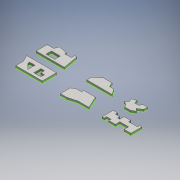
# Autodesk Inventor part: 240329_직선연습
Saved by Autodesk Inventor 2016 (Build 200138000, 138)
## iProperties
Created: 2024-03-29
Part Number: 240329_직선연습
Material: 일반
Document SubType Name: Modeling
Designer: pc
Density: 1 g/cm^3
Appearance: 기본값
Author: pc
Autodesk Inventor part; units mm, degrees
ref_plane "YZ Plane" through (0, 0, 0) normal (1, 0, 0) x (0, 1, 0)
ref_plane "XZ Plane" through (0, 0, 0) normal (0, 1, 0) x (-1, 0, 0)
ref_plane "XY Plane" through (0, 0, 0) normal (0, 0, 1) x (1, 0, 0)
sketch "스케치1" plane through (0, 0, 0) normal (0, 0, 1) x (1, 0, 0)
  line L0 (-17.9838, 5.9383) -> (12.0162, 5.9383)
  line L1 (-17.9838, 5.9383) -> (-17.9838, -44.0617)
  line L2 (-17.9838, -44.0617) -> (110.0162, -44.0617)
  line L3 (110.0162, -44.0617) -> (97.8609, 24.8748)
  line L4 (97.8609, 24.8748) -> (87.8609, 24.8748)
  line L5 (87.8609, 24.8748) -> (87.8609, 9.8748)
  line L6 (87.8609, 9.8748) -> (57.8609, 9.8748)
  line L7 (57.8609, 9.8748) -> (57.8609, 17.8748)
  line L8 (57.8609, 17.8748) -> (18.4685, 24.8207)
  line L9 (18.4685, 24.8207) -> (12.0162, 5.9383)
  line L10 (17.0386, -9.366) -> (57.0386, -9.366)
  line L11 (57.0386, -9.366) -> (57.0386, -34.366)
  line L12 (57.0386, -34.366) -> (17.0386, -34.366)
  line L13 (17.0386, -34.366) -> (17.0386, -9.366)
  line L14 (-21.4983, -83.6189) -> (113.5017, -83.6189)
  line L15 (113.5017, -83.6189) -> (113.5017, -147.6189)
  line L16 (113.5017, -147.6189) -> (-6.4983, -147.6189)
  line L17 (-6.4983, -147.6189) -> (-6.4983, -112.6189)
  line L18 (-6.4983, -112.6189) -> (-21.4983, -83.6189)
  line L19 (11.4782, -102.6977) -> (11.4782, -110.6977)
  line L20 (11.4782, -102.6977) -> (35.4782, -102.6977)
  line L21 (35.4782, -102.6977) -> (35.4782, -134.6977)
  line L22 (35.4782, -134.6977) -> (11.4782, -110.6977)
  line L23 (62.4782, -102.6977) -> (62.4782, -134.6977)
  line L24 (62.4782, -134.6977) -> (94.4782, -134.6977)
  line L25 (94.4782, -134.6977) -> (94.4782, -118.6977)
  line L26 (94.4782, -118.6977) -> (78.4782, -118.6977)
  line L27 (78.4782, -118.6977) -> (78.4782, -102.6977)
  line L28 (78.4782, -102.6977) -> (62.4782, -102.6977)
  line L29 (210.3042, -22.2898) -> (210.3042, -42.2898)
  line L30 (210.3042, -42.2898) -> (325.3042, -42.2898)
  line L31 (325.3042, -42.2898) -> (308.521, -17.4237)
  line L32 (308.521, -17.4237) -> (288.521, -17.4237)
  line L33 (288.521, -17.4237) -> (279.9747, 2.7102)
  line L34 (279.9747, 2.7102) -> (240.098, 2.7102)
  line L35 (240.098, 2.7102) -> (210.3042, -22.2898)
  line L36 (243.03, -90.9913) -> (298.03, -90.9913)
  line L37 (298.03, -90.9913) -> (323.3871, -145.3698)
  line L38 (323.3871, -145.3698) -> (273.3871, -145.3698)
  line L39 (273.3871, -145.3698) -> (234.8117, -156.4311)
  line L40 (234.8117, -156.4311) -> (204.822, -156.4311)
  line L41 (204.822, -156.4311) -> (204.822, -111.4311)
  line L42 (204.822, -111.4311) -> (222.1425, -101.4311)
  line L43 (222.1425, -101.4311) -> (247.0375, -101.4311)
  line L44 (247.0375, -101.4311) -> (243.03, -90.9913)
  line L45 (391.7462, -29.9278) -> (380.8188, -42.9505)
  line L46 (380.8188, -42.9505) -> (394.4134, -49.2898)
  line L47 (394.4134, -49.2898) -> (404.1642, -63.2154)
  line L48 (404.1642, -63.2154) -> (429.1642, -63.2154)
  line L49 (429.1642, -63.2154) -> (446.4847, -53.2154)
  line L50 (391.7462, -29.9278) -> (386.6159, -15.8324)
  line L51 (391.7462, -29.9278) -> (406.7462, -29.9278) construction
  line L52 (386.6159, -15.8324) -> (405.4097, -8.992)
  line L53 (405.4097, -8.992) -> (411.2241, -24.9667)
  line L54 (455.4729, -12.2341) -> (435.4737, -12.0471)
  line L55 (435.4737, -12.0471) -> (427.8526, -24.9667)
  line L56 (411.2241, -24.9667) -> (427.8526, -24.9667)
  line L57 (455.4729, -12.2341) -> (455.4729, -29.2341)
  line L58 (455.4729, -29.2341) -> (434.9941, -43.5735)
  line L59 (434.9941, -43.5735) -> (446.4847, -53.2154)
  line L60 (390.4902, -102.3026) -> (410.4902, -102.3026)
  line L61 (410.4902, -102.3026) -> (410.4902, -112.3026)
  line L62 (410.4902, -112.3026) -> (430.4902, -112.3026)
  line L63 (430.4902, -112.3026) -> (430.4902, -122.3026)
  line L64 (430.4902, -122.3026) -> (440.4902, -122.3026)
  line L65 (440.4902, -122.3026) -> (440.4902, -102.3026)
  line L66 (440.4902, -102.3026) -> (470.4902, -102.3026)
  line L67 (470.4902, -102.3026) -> (470.4902, -112.3026)
  line L68 (470.4902, -112.3026) -> (510.4902, -112.3026)
  line L69 (510.4902, -112.3026) -> (510.4902, -102.3026)
  line L70 (510.4902, -102.3026) -> (520.4902, -102.3026)
  line L71 (520.4902, -102.3026) -> (520.4902, -152.3026)
  line L72 (390.4902, -102.3026) -> (390.4902, -152.3026)
  line L73 (390.4902, -152.3026) -> (400.4902, -152.3026)
  line L74 (400.4902, -152.3026) -> (400.4902, -142.3026)
  line L75 (400.4902, -142.3026) -> (420.4902, -142.3026)
  line L76 (420.4902, -142.3026) -> (420.4902, -152.3026)
  line L77 (420.4902, -152.3026) -> (450.4902, -152.3026)
  line L78 (450.4902, -152.3026) -> (450.4902, -132.3026)
  line L79 (450.4902, -132.3026) -> (490.4902, -132.3026)
  line L80 (490.4902, -132.3026) -> (490.4902, -152.3026)
  line L81 (490.4902, -152.3026) -> (520.4902, -152.3026)
  point P0 (0, 0)
  dimension "d0" = 30
  dimension "d1" = 50
  dimension "d2" = 128
  dimension "d3" = 70
  dimension "d4" = 80
  dimension "d5" = 10
  dimension "d6" = 15
  dimension "d7" = 30
  dimension "d8" = 8
  dimension "d9" = 40
  dimension "d10" = 100
  dimension "d11" = 40
  dimension "d12" = 25
  dimension "d13" = 135
  dimension "d14" = 64
  dimension "d15" = 120
  dimension "d16" = 35
  dimension "d17" = 8
  dimension "d18" = 24
  dimension "d19" = 32
  dimension "d20" = 32
  dimension "d21" = 16
  dimension "d22" = 16
  dimension "d23" = 27
  dimension "d28" = 20
  dimension "d29" = 115
  dimension "d30" = 30
  dimension "d31" = 20
  dimension "d32" = 67
  dimension "d33" = 50
  dimension "d34" = 45
  dimension "d35" = 55
  dimension "d36" = 60
  dimension "d37" = 50
  dimension "d38" = 65
  dimension "d39" = 40.13
  dimension "d40" = 16
  dimension "d41" = 45
  dimension "d42" = 20
  dimension "d43" = 120
  dimension "d44" = 69
  dimension "d56" = 17
  dimension "d58" = 15
  dimension "d59" = 75
  dimension "d60" = 17
  dimension "d61" = 150
  dimension "d62" = 25
  dimension "d63" = 20
  dimension "d64" = 150
  dimension "d77" = 125
  dimension "d78" = 15
  dimension "d80" = 20
  dimension "d81" = 17
  dimension "d82" = 20
  dimension "d83" = 15
  dimension "d84" = 120
  dimension "d85" = 120
  dimension "d87" = 90
  dimension "d88" = 90
  dimension "d97" = 17
  dimension "d98" = 25
  dimension "d99" = 55
  dimension "d100" = 75
  dimension "d103" = 20
  constraints: 164 end point, 33 perpendicular, 10 horizontal, 8 vertical, 7 point on line, 4 parallel
  measures "d0" distance of L0.start L0.end
  measures "d1" distance of L0.start L1.end
  measures "d2" distance of L1.end L2.end
  measures "d3" distance of L2.end L3.end
  measures "d4" angle of L3 L2
  measures "d5" distance of L3.end L4.end
  measures "d6" distance of L4.end L5.end
  measures "d7" distance of L5.end L6.end
  measures "d8" distance of L6.end L7.end
  measures "d9" distance of L7.end L8.end
  measures "d10" angle of L8 L7
  measures "d11" distance of L11.end L12.end
  measures "d12" distance of L10.end L11.end
  measures "d13" distance of L14.start L14.end
  measures "d14" distance of L14.end L15.end
  measures "d15" distance of L15.end L16.end
  measures "d16" distance of L16.end L17.end
  measures "d17" distance of L19.start L19.end
  measures "d18" distance of L19.start L20.end
  measures "d19" distance of L20.end L21.end
  measures "d20" distance of L23.end L24.end
  measures "d21" distance of L25.end L26.end
  measures "d22" distance of L26.end L27.end
  measures "d23" distance of L23.start L20.end
  measures "d28" distance of L29.start L29.end
  measures "d29" distance of L29.end L30.end
  measures "d30" distance of L30.end L31.end
  measures "d31" distance of L31.end L32.end
  measures "d32" angle of L32 L33
  measures "d33" angle of L29 L35
  measures "d34" distance between parallel lines of L30 L34
  measures "d35" distance of L36.start L36.end
  measures "d36" distance of L36.end L37.end
  measures "d37" distance of L37.end L38.end
  measures "d38" angle of L37 L38
  measures "d39" distance of L38.end L39.end
  measures "d40" angle of L40 L39
  measures "d41" distance of L40.end L41.end
  measures "d42" distance of L41.end L42.end
  measures "d43" angle of L41 L42
  measures "d44" angle of L44 L43
  measures "d56" distance of L45.start L45.end
  measures "d58" distance of L45.end L46.end
  measures "d59" angle of L46 L45
  measures "d60" distance of L46.end L47.end
  measures "d61" angle of L46 L47
  measures "d62" distance of L47.end L48.end
  measures "d63" distance of L48.end L49.end
  measures "d64" angle of L49 L48
  measures "d77" angle of L48 L47
  measures "d78" distance of L45.start L50.end
  measures "d80" distance of L50.end L52.end
  measures "d81" distance of L52.end L53.end
  measures "d82" distance of L54.start L54.end
  measures "d83" distance of L54.end L55.end
  measures "d84" angle of L55 L54
  measures "d85" angle of L45 L50
  measures "d87" angle of L53 L52
  measures "d88" angle of L50 L52
  measures "d97" distance of L54.start L57.end
  measures "d98" distance of L57.end L58.end
  measures "d99" angle of L57 L58
  measures "d100" angle of L59 L58
  measures "d103" distance of L60.start L60.end
extrude "돌출1" add sketch "스케치1" along normal blind 10 contours L0 L9 L8 L7 L6 L5 L4 L3 L2 L1
extrude "돌출2" add sketch "스케치1" along normal blind 10 contours L14 L15 L16 L17 L18
extrude "돌출3" add sketch "스케치1" along normal blind 10 contours L35 L34 L33 L32 L31 L30 L29
extrude "돌출4" add sketch "스케치1" along normal blind 10 contours L36 L37 L38 L39 L40 L41 L42 L43 L44
extrude "돌출5" add sketch "스케치1" along normal blind 10 contours L50 L52 L53 L56 L55 L54 L57 L58 L59 L49 L48 L47 L46 L45
extrude "돌출6" add sketch "스케치1" along normal blind 10 contours L60 L61 L62 L63 L64 L65 L66 L67 L68 L69 L70 L71 L81 L80 L79 L78 L77 L76 L75 L74 L73 L72
